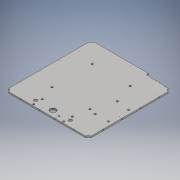
# Autodesk Inventor part: 001
Saved by Autodesk Inventor 2016 (Build 200138000, 138)
## iProperties
Created: 2015-10-17
Part Number: 001
Material: Generic
Document SubType Name: Modeling
Designer: iLyngklip
Density: 1 g/cm^3
Appearance: Default
Author: iLyngklip
Title: Mellemplade mk2
Autodesk Inventor part; units mm, degrees
ref_plane "YZ Plane" through (0, 0, 0) normal (1, 0, 0) x (0, 1, 0)
ref_plane "XZ Plane" through (0, 0, 0) normal (0, 1, 0) x (-1, 0, 0)
ref_plane "XY Plane" through (0, 0, 0) normal (0, 0, 1) x (1, 0, 0)
sketch "Sketch1" plane through (0, 0, 0) normal (0, 0, 1) x (1, 0, 0)
  line L0 (-154, 160) -> (154, 160)
  line L1 (154, 160) -> (154, -160)
  line L2 (154, -160) -> (-154, -160)
  line L3 (-154, -160) -> (-154, 160)
  point P0 (0, 0)
  dimension "d0" = 308
  dimension "d1" = 320
  dimension "d2" = 160
  dimension "d3" = 154
  constraints: 8 end point, 2 parallel, 1 horizontal, 1 perpendicular
  measures "d0" distance of L1.end L2.end
  measures "d1" distance of L0.end L1.end
  measures "d2" distance from line of L0 point (0, 0)
  measures "d3" distance from line of point (0, 0) L1
extrude "Tykkelse" add sketch "Sketch1" along normal blind 6
sketch "Sketch2" plane through (0, 0, 6) normal (0, 0, 1) x (1, 0, 0)
  circle A0 centre (65, -138) radius 6
  circle A1 centre (-65, -138) radius 6
  circle A2 centre (0, -138) radius 11
  line L0 (0, 0) -> (0, -168.7414) construction
  line L1 (-154, -160) -> (154, -160) projected
  line L2 (154, -160) -> (154, 160) projected
  dimension "d7" = 12
  dimension "d8" = 22
  dimension "d9" = 22
  dimension "d10" = 130
  dimension "d15" = 22
  dimension "d16" = 22
  dimension "d135" = 12
  dimension "d136" = 89
  constraints: 3 centre point, 2 end point, 1 point on line, 1 vertical
  measures "d7" diameter of A0
  measures "d8" diameter of A2
  measures "d9" distance from line of L1 A0.centre
  measures "d10" distance of A0.centre A1.centre
  measures "d15" distance from line of L1 A2.centre
  measures "d16" distance from line of L1 A1.centre
  measures "d135" diameter of A1
  measures "d136" distance from line of L2 A0.centre
extrude "Ø12 Glide hul" cut sketch "Sketch2" against normal blind 3 contours A0 | A1
extrude "Gevind hul" cut sketch "Sketch2" against normal blind 6 contours A2
sketch "Sketch3" plane through (0, 0, 6) normal (0, 0, 1) x (1, 0, 0)
  circle A0 centre (154, -160) radius 10
  line L0 (154, -160) -> (-154, -160) projected
  circle A1 centre (-154, -160) radius 10
  line L1 (154, 160) -> (-154, 160) projected
  circle A2 centre (154, 160) radius 11.5178
  circle A3 centre (-154, 160) radius 10
  point P0 (0, 0)
  dimension "d17" = 20
  dimension "d18" = 20
  dimension "d21" = 20
  dimension "d22" = 23.0357
  constraints: 4 centre point, 2 coincident
  measures "d17" diameter of A0
  measures "d18" diameter of A1
  measures "d21" diameter of A3
  measures "d22" diameter of A2
extrude "Ledningsrunding" cut sketch "Sketch3" against normal blind 10
sketch "Sketch4" plane through (0, 0, 0) normal (0, 0, -1) x (-1, 0, 0)
  circle A0 centre (56.15, -121.85) radius 1.5 projected
  circle A1 centre (56.15, -154.15) radius 1.5 projected
  circle A2 centre (-56.15, -154.15) radius 1.5 projected
  circle A3 centre (-56.15, -121.85) radius 1.5 projected
  point P0 (0, 0)
extrude "Step-spacer montering" cut sketch "Sketch4" against normal up to surface (6 mm away)
sketch "Sketch5" plane through (0, 0, 0) normal (0, 0, -1) x (-1, 0, 0)
  circle A0 centre (77, 85) radius 1.5
  circle A1 centre (77, -65) radius 1.5
  circle A2 centre (-65, -65) radius 1.5
  circle A3 centre (-65, 85) radius 1.5
  point P0 (0, 0)
  dimension "d119" = 3
  dimension "d120" = 150
  dimension "d121" = 142
  dimension "d122" = 85
  dimension "d123" = 65
  constraints: 4 centre point, 3 equal radius, 2 horizontal alignment, 2 vertical alignment
  measures "d119" diameter of A0
  measures "d120" distance of A1.centre A0.centre
  measures "d121" distance of A2.centre A1.centre
  measures "d122" vertical distance of point (0, 0) A0.centre
  measures "d123" horizontal distance of point (0, 0) A2.centre
extrude "PSU-Mount holes" cut sketch "Sketch5" against normal up to surface (6 mm away)
sketch "Sketch6" plane through (0, 0, 0) normal (0, 0, -1) x (-1, 0, 0)
  circle A0 centre (-90.74, -71.27) radius 1.5875 projected
  circle A1 centre (-139, -70) radius 1.5875 projected
  circle A2 centre (-139, 4.93) radius 1.5875 projected
  circle A3 centre (-90.74, 11.28) radius 1.5875 projected
  point P0 (0, 0)
extrude "Ramps Mount holes" cut sketch "Sketch6" against normal up to surface (6 mm away)
sketch "Sketch7" plane through (0, 0, 6) normal (0, 0, 1) x (1, 0, 0)
  line L0 (142.4822, 160) -> (-144, 160) projected
  line L1 (58.5, 160) -> (151.5, 160)
  line L2 (151.5, 160) -> (151.5, 152)
  line L3 (151.5, 152) -> (58.5, 152)
  line L4 (58.5, 152) -> (58.5, 160)
  line L5 (144.5, 166) -> (65.5, 166) projected
  line L6 (130.5, 152) -> (151.5, 152)
  line L7 (151.5, 152) -> (151.5, 148)
  line L8 (151.5, 148) -> (130.5, 148)
  line L9 (130.5, 148) -> (130.5, 152)
  line L10 (151.5, 148) -> (160.3981, 148)
  line L11 (160.3981, 148) -> (160.3981, 160)
  line L12 (160.3981, 160) -> (151.5, 160)
  line L13 (151.5, 160) -> (151.5, 148)
  point P0 (0, 0)
  dimension "d29" = 14
  dimension "d30" = 93
  dimension "d31" = 79
  dimension "d33" = 7
  dimension "d36" = 4
  dimension "d37" = 21
  constraints: 24 end point, 6 parallel, 3 horizontal, 3 perpendicular, 2 point on line
  measures "d29" distance between parallel lines of L3 L5
  measures "d30" distance of L2.end L3.end
  measures "d31" distance of L5.start L5.end
  measures "d33" horizontal distance of L5.end L3.end
  measures "d36" distance of L6.end L7.end
  measures "d37" distance of L7.end L8.end
extrude "Skærm-plads" cut sketch "Sketch7" against normal up to next
sketch "Sketch8" plane through (0, 0, 0) normal (0, 0, -1) x (-1, 0, 0)
  line L0 (-58.5, 160) -> (-58.5, 152) construction
  line L1 (-58.5, 152) -> (-130.5, 152) construction
  line L2 (-130.5, 152) -> (-130.5, 148) construction
  line L3 (-130.5, 148) -> (-154, 148) construction
  line L4 (-154, 148) -> (-154, -150) construction
  arc A0 (-144, -160) -> (-154, -150) centre (-154, -160) ccw construction
  line L5 (-144, -160) -> (144, -160) construction
  arc A1 (154, -150) -> (144, -160) centre (154, -160) ccw construction
  line L6 (154, -150) -> (154, 150) projected
  arc A2 (144, 160) -> (154, 150) centre (154, 160) ccw construction
  line L7 (144, 160) -> (-58.5, 160) projected
  circle A3 centre (0, -138) radius 11 construction
  circle A4 centre (56.15, -121.85) radius 1.5 construction
  circle A5 centre (56.15, -154.15) radius 1.5 construction
  circle A6 centre (-56.15, -121.85) radius 1.5 construction
  circle A7 centre (-56.15, -154.15) radius 1.5 construction
  circle A8 centre (-90.74, -71.27) radius 1.5875 construction
  circle A9 centre (-139, -70) radius 1.5875 construction
  circle A10 centre (-90.74, 11.28) radius 1.5875 construction
  circle A11 centre (-139, 4.93) radius 1.5875 construction
  line L8 (154, 103.5) -> (147.679, 103.5)
  line L9 (147.679, 103.5) -> (147.679, 103.5)
  line L10 (146.179, 102) -> (144.779, 102)
  line L11 (144.779, 108) -> (146.179, 108)
  line L12 (147.679, 106.5) -> (147.679, 106.5)
  line L13 (147.679, 106.5) -> (154, 106.5)
  arc A12 (146.179, 102) -> (147.679, 103.5) centre (146.179, 103.5) ccw
  arc A13 (147.679, 106.5) -> (146.179, 108) centre (146.179, 106.5) ccw
  arc A14 (143.279, 103.5) -> (144.779, 102) centre (144.779, 103.5) ccw
  arc A15 (143.279, 106.5) -> (143.279, 103.5) centre (143.279, 105) ccw
  arc A16 (143.279, 106.5) -> (142.4708, 103.7364) centre (143.279, 105) ccw
  arc A17 (144.779, 108) -> (143.279, 106.5) centre (144.779, 106.5) ccw
  line L14 (143.279, 105) -> (153.6341, 105) construction
  arc A18 (146.179, 32) -> (147.679, 33.5) centre (146.179, 33.5) ccw
  arc A19 (143.279, 33.5) -> (144.779, 32) centre (144.779, 33.5) ccw
  line L15 (146.179, 32) -> (144.779, 32)
  line L16 (154, 33.5) -> (147.679, 33.5)
  line L17 (147.679, 33.5) -> (147.679, 33.5)
  line L18 (147.679, 36.5) -> (154, 36.5)
  line L19 (147.679, 36.5) -> (147.679, 36.5)
  arc A20 (147.679, 36.5) -> (146.179, 38) centre (146.179, 36.5) ccw
  line L20 (143.279, 35) -> (153.6341, 35) construction
  line L21 (144.779, 38) -> (146.179, 38)
  arc A21 (143.279, 36.5) -> (143.279, 33.5) centre (143.279, 35) ccw
  arc A22 (143.279, 36.5) -> (142.4708, 33.7364) centre (143.279, 35) ccw
  arc A23 (144.779, 38) -> (143.279, 36.5) centre (144.779, 36.5) ccw
  arc A24 (146.179, -38) -> (147.679, -36.5) centre (146.179, -36.5) ccw
  arc A25 (143.279, -36.5) -> (144.779, -38) centre (144.779, -36.5) ccw
  line L22 (146.179, -38) -> (144.779, -38)
  line L23 (154, -36.5) -> (147.679, -36.5)
  line L24 (147.679, -36.5) -> (147.679, -36.5)
  line L25 (147.679, -33.5) -> (154, -33.5)
  line L26 (147.679, -33.5) -> (147.679, -33.5)
  arc A26 (147.679, -33.5) -> (146.179, -32) centre (146.179, -33.5) ccw
  line L27 (143.279, -35) -> (153.6341, -35) construction
  line L28 (144.779, -32) -> (146.179, -32)
  arc A27 (143.279, -33.5) -> (143.279, -36.5) centre (143.279, -35) ccw
  arc A28 (143.279, -33.5) -> (142.4708, -36.2636) centre (143.279, -35) ccw
  arc A29 (144.779, -32) -> (143.279, -33.5) centre (144.779, -33.5) ccw
  arc A30 (146.179, -108) -> (147.679, -106.5) centre (146.179, -106.5) ccw
  arc A31 (143.279, -106.5) -> (144.779, -108) centre (144.779, -106.5) ccw
  line L29 (146.179, -108) -> (144.779, -108)
  line L30 (154, -106.5) -> (147.679, -106.5)
  line L31 (147.679, -106.5) -> (147.679, -106.5)
  line L32 (147.679, -103.5) -> (154, -103.5)
  line L33 (147.679, -103.5) -> (147.679, -103.5)
  arc A32 (147.679, -103.5) -> (146.179, -102) centre (146.179, -103.5) ccw
  line L34 (143.279, -105) -> (153.6341, -105) construction
  line L35 (144.779, -102) -> (146.179, -102)
  arc A33 (143.279, -103.5) -> (143.279, -106.5) centre (143.279, -105) ccw
  arc A34 (143.279, -103.5) -> (142.4708, -106.2636) centre (143.279, -105) ccw
  arc A35 (144.779, -102) -> (143.279, -103.5) centre (144.779, -103.5) ccw
  line L36 (144, -160) -> (-144, -160) projected
  line L37 (100.5, -160) -> (100.5, -153.679)
  line L38 (97.5, -160) -> (97.5, -153.679)
  arc A36 (100.5, -149.279) -> (97.5, -149.279) centre (99, -149.279) ccw
  arc A37 (96, -152.179) -> (97.5, -153.679) centre (97.5, -152.179) ccw
  line L39 (96, -152.179) -> (96, -150.779)
  arc A38 (97.5, -149.279) -> (96, -150.779) centre (97.5, -150.779) ccw
  arc A39 (100.5, -153.679) -> (102, -152.179) centre (100.5, -152.179) ccw
  line L40 (102, -152.179) -> (102, -150.779)
  arc A40 (102, -150.779) -> (100.5, -149.279) centre (100.5, -150.779) ccw
  line L41 (26, -152.179) -> (26, -150.779)
  arc A41 (27.5, -149.279) -> (26, -150.779) centre (27.5, -150.779) ccw
  arc A42 (26, -152.179) -> (27.5, -153.679) centre (27.5, -152.179) ccw
  arc A43 (30.5, -149.279) -> (27.5, -149.279) centre (29, -149.279) ccw
  line L42 (27.5, -160) -> (27.5, -153.679)
  arc A44 (32, -150.779) -> (30.5, -149.279) centre (30.5, -150.779) ccw
  line L43 (32, -152.179) -> (32, -150.779)
  arc A45 (30.5, -153.679) -> (32, -152.179) centre (30.5, -152.179) ccw
  line L44 (30.5, -160) -> (30.5, -153.679)
  line L45 (99, -149.279) -> (99, -156.2509) construction
  line L46 (-67.1744, 0) -> (89.9011, 0) construction
  line L47 (0, -73.7565) -> (0, 76.0519) construction
  line L48 (100.5, 160) -> (100.5, 153.679)
  line L49 (97.5, 160) -> (97.5, 153.679)
  arc A46 (97.5, 149.279) -> (100.5, 149.279) centre (99, 149.279) ccw
  arc A47 (97.5, 153.679) -> (96, 152.179) centre (97.5, 152.179) ccw
  line L50 (96, 152.179) -> (96, 150.779)
  arc A48 (96, 150.779) -> (97.5, 149.279) centre (97.5, 150.779) ccw
  arc A49 (102, 152.179) -> (100.5, 153.679) centre (100.5, 152.179) ccw
  line L51 (102, 152.179) -> (102, 150.779)
  arc A50 (100.5, 149.279) -> (102, 150.779) centre (100.5, 150.779) ccw
  line L52 (99, 149.279) -> (99, 156.2509) construction
  arc A51 (-1.5, 149.279) -> (1.5, 149.279) centre (0, 149.279) ccw
  arc A52 (-3, 150.779) -> (-1.5, 149.279) centre (-1.5, 150.779) ccw
  arc A53 (1.5, 149.279) -> (3, 150.779) centre (1.5, 150.779) ccw
  line L53 (-3, 152.179) -> (-3, 150.779)
  line L54 (3, 152.179) -> (3, 150.779)
  arc A54 (-1.5, 153.679) -> (-3, 152.179) centre (-1.5, 152.179) ccw
  arc A55 (3, 152.179) -> (1.5, 153.679) centre (1.5, 152.179) ccw
  line L55 (0, 149.279) -> (0, 156.2509) construction
  line L56 (-1.5, 160) -> (-1.5, 153.679)
  line L57 (1.5, 160) -> (1.5, 153.679)
  arc A56 (-147.679, 33.5) -> (-146.179, 32) centre (-146.179, 33.5) ccw
  arc A57 (-144.779, 32) -> (-143.279, 33.5) centre (-144.779, 33.5) ccw
  line L58 (-146.179, 32) -> (-144.779, 32)
  line L59 (-154, 33.5) -> (-147.679, 33.5)
  line L60 (-147.679, 33.5) -> (-147.679, 33.5)
  line L61 (-147.679, 36.5) -> (-154, 36.5)
  line L62 (-147.679, 36.5) -> (-147.679, 36.5)
  arc A58 (-146.179, 38) -> (-147.679, 36.5) centre (-146.179, 36.5) ccw
  line L63 (-143.279, 35) -> (-153.6341, 35) construction
  line L64 (-144.779, 38) -> (-146.179, 38)
  arc A59 (-143.279, 33.5) -> (-143.279, 36.5) centre (-143.279, 35) ccw
  arc A60 (-142.4708, 33.7364) -> (-143.279, 36.5) centre (-143.279, 35) ccw
  arc A61 (-143.279, 36.5) -> (-144.779, 38) centre (-144.779, 36.5) ccw
  arc A62 (-143.279, -36.5) -> (-143.279, -33.5) centre (-143.279, -35) ccw
  arc A63 (-142.4708, -36.2636) -> (-143.279, -33.5) centre (-143.279, -35) ccw
  arc A64 (-144.779, -38) -> (-143.279, -36.5) centre (-144.779, -36.5) ccw
  line L65 (-144.779, -32) -> (-146.179, -32)
  arc A65 (-143.279, -33.5) -> (-144.779, -32) centre (-144.779, -33.5) ccw
  line L66 (-146.179, -38) -> (-144.779, -38)
  arc A66 (-147.679, -36.5) -> (-146.179, -38) centre (-146.179, -36.5) ccw
  line L67 (-147.679, -36.5) -> (-147.679, -36.5)
  line L68 (-147.679, -33.5) -> (-147.679, -33.5)
  arc A67 (-146.179, -32) -> (-147.679, -33.5) centre (-146.179, -33.5) ccw
  line L69 (-143.279, -35) -> (-153.6341, -35) construction
  line L70 (-154, -36.5) -> (-147.679, -36.5)
  line L71 (-147.679, -33.5) -> (-154, -33.5)
  arc A68 (-143.279, -106.5) -> (-143.279, -103.5) centre (-143.279, -105) ccw
  arc A69 (-142.4708, -106.2636) -> (-143.279, -103.5) centre (-143.279, -105) ccw
  arc A70 (-144.779, -108) -> (-143.279, -106.5) centre (-144.779, -106.5) ccw
  line L72 (-144.779, -102) -> (-146.179, -102)
  arc A71 (-143.279, -103.5) -> (-144.779, -102) centre (-144.779, -103.5) ccw
  line L73 (-146.179, -108) -> (-144.779, -108)
  arc A72 (-147.679, -106.5) -> (-146.179, -108) centre (-146.179, -106.5) ccw
  line L74 (-147.679, -106.5) -> (-147.679, -106.5)
  line L75 (-147.679, -103.5) -> (-147.679, -103.5)
  arc A73 (-146.179, -102) -> (-147.679, -103.5) centre (-146.179, -103.5) ccw
  line L76 (-143.279, -105) -> (-153.6341, -105) construction
  line L77 (-154, -106.5) -> (-147.679, -106.5)
  line L78 (-147.679, -103.5) -> (-154, -103.5)
  line L79 (-100.5, -160) -> (-100.5, -153.679)
  line L80 (-97.5, -160) -> (-97.5, -153.679)
  arc A74 (-97.5, -149.279) -> (-100.5, -149.279) centre (-99, -149.279) ccw
  arc A75 (-97.5, -153.679) -> (-96, -152.179) centre (-97.5, -152.179) ccw
  line L81 (-96, -152.179) -> (-96, -150.779)
  arc A76 (-96, -150.779) -> (-97.5, -149.279) centre (-97.5, -150.779) ccw
  arc A77 (-102, -152.179) -> (-100.5, -153.679) centre (-100.5, -152.179) ccw
  line L82 (-102, -152.179) -> (-102, -150.779)
  arc A78 (-100.5, -149.279) -> (-102, -150.779) centre (-100.5, -150.779) ccw
  line L83 (-26, -152.179) -> (-26, -150.779)
  arc A79 (-26, -150.779) -> (-27.5, -149.279) centre (-27.5, -150.779) ccw
  arc A80 (-27.5, -153.679) -> (-26, -152.179) centre (-27.5, -152.179) ccw
  arc A81 (-27.5, -149.279) -> (-30.5, -149.279) centre (-29, -149.279) ccw
  line L84 (-27.5, -160) -> (-27.5, -153.679)
  arc A82 (-30.5, -149.279) -> (-32, -150.779) centre (-30.5, -150.779) ccw
  line L85 (-32, -152.179) -> (-32, -150.779)
  arc A83 (-32, -152.179) -> (-30.5, -153.679) centre (-30.5, -152.179) ccw
  line L86 (-30.5, -160) -> (-30.5, -153.679)
  line L87 (-99, -149.279) -> (-99, -156.2509) construction
  line L88 (-154, -150) -> (-154, 148.4822) projected
  line L89 (-154, 103.5) -> (-147.679, 103.5)
  line L90 (-154, 106.4661) -> (-147.679, 106.4661)
  arc A84 (-147.679, 103.5) -> (-146.1791, 102) centre (-146.179, 103.5) ccw
  line L91 (-146.1791, 102) -> (-144.7791, 102)
  arc A85 (-144.7791, 102) -> (-143.2791, 103.5) centre (-144.7791, 103.5) ccw
  arc A86 (-143.2791, 103.5) -> (-143.2791, 106.5) centre (-143.2791, 105) ccw
  arc A87 (-143.2791, 106.5) -> (-144.7787, 107.9661) centre (-144.7787, 106.4661) ccw
  arc A88 (-146.1787, 107.9661) -> (-147.679, 106.4661) centre (-146.179, 106.4661) ccw
  line L92 (-146.1787, 107.9661) -> (-144.7787, 107.9661)
  line L93 (-143.2791, 105) -> (-148.8776, 105) construction
  line L94 (154, 106.5) -> (154, 103.5)
  line L95 (154, 36.5) -> (154, 33.5)
  line L96 (154, 150) -> (154, -150) projected
  line L97 (154, -33.5) -> (154, -36.5)
  line L98 (154, -103.5) -> (154, -106.5)
  line L99 (100.5, -160) -> (97.5, -160)
  line L100 (30.5, -160) -> (27.5, -160)
  line L101 (-27.5, -160) -> (-30.5, -160)
  line L102 (-97.5, -160) -> (-100.5, -160)
  line L103 (-154, -106.5) -> (-154, -103.5)
  line L104 (-154, -36.5) -> (-154, -33.5)
  line L105 (-154, 33.5) -> (-154, 36.5)
  line L106 (-154, 103.5) -> (-154, 106.4661)
  line L107 (100.5, 160) -> (97.5, 160)
  line L108 (144, 160) -> (-58.5, 160) projected
  line L109 (1.5, 160) -> (-1.5, 160)
  point P0 (0, 0)
  point P1 (147.679, 106.5)
  point P2 (143.279, 33.5)
  point P3 (147.679, 36.5)
  point P4 (147.679, -33.5)
  point P5 (147.679, -103.5)
  point P6 (-143.279, 33.5)
  point P7 (-147.679, 36.5)
  point P8 (-143.279, -36.5)
  point P9 (-147.679, -33.5)
  point P10 (-147.679, -103.5)
  dimension "d38" = 6.321
  dimension "d40" = 1.5
  dimension "d41" = 1.4
  dimension "d42" = 1.5
  dimension "d43" = 1.5
  dimension "d44" = 1.4
  dimension "d45" = 55
  dimension "d48" = 70
  dimension "d56" = 1.5
  dimension "d57" = 1.4
  dimension "d58" = 1.5
  dimension "d59" = 6.321
  dimension "d60" = 1.5
  dimension "d61" = 1.4
  dimension "d62" = 1.5
  dimension "d63" = 1.5
  dimension "d66" = 70
  dimension "d71" = 55
  dimension "d74" = 99
  dimension "d81" = 70
  dimension "d86" = 1.5
  dimension "d87" = 1.4
  dimension "d88" = 6.321
  dimension "d91" = 55
  constraints: 203 end point, 160 point on circle, 77 centre point, 70 symmetric about line, 27 point on line, 21 coincident, 16 vertical, 12 collinear, 12 horizontal alignment, 11 tangent, 10 perpendicular, 9 horizontal, 7 equal radius, 7 vertical alignment, 4 parallel, 1 midpoint, 281 other
  measures "d38" distance of L8.start L8.end
  measures "d40" radius of A12
  measures "d41" distance of L11.start L11.end
  measures "d42" radius of A15
  measures "d43" radius of A17
  measures "d44" distance of A17.centre A13.centre
  measures "d45" distance between parallel lines of L7 L14
  measures "d48" distance of A12.centre A18.centre
  measures "d56" radius of A37
  measures "d57" distance of L39.start L39.end
  measures "d58" radius of A38
  measures "d59" distance of L38.start L38.end
  measures "d60" radius of A39
  measures "d61" distance of L40.start L40.end
  measures "d62" radius of A40
  measures "d63" radius of A36
  measures "d66" distance of L39.start L41.start
  measures "d71" distance between parallel lines of L6 L45
  measures "d74" distance of L52.start L55.start
  measures "d81" distance of A60.start A63.start
  measures "d86" radius of A88
  measures "d87" distance of L91.start L91.end
  measures "d88" distance of L89.start L89.end
  measures "d91" distance between parallel lines of L7 L93
extrude "Monteringshuller" cut sketch "Sketch8" against normal blind 5
sketch "Sketch10" plane through (0, 0, 6) normal (0, 0, 1) x (1, 0, 0)
  line L0 (58.5, 152) -> (58.5, 160) projected
  line L1 (58.5, 160) -> (-144, 160) projected
  arc A0 (-154, 150) -> (-144, 160) centre (-154, 160) ccw projected
  line L2 (-154, 150) -> (-154, -150) projected
  arc A1 (-144, -160) -> (-154, -150) centre (-154, -160) ccw projected
  line L3 (-144, -160) -> (144, -160) projected
  arc A2 (154, -150) -> (144, -160) centre (154, -160) ccw projected
  line L4 (154, -150) -> (154, 148) projected
  line L5 (154, 148) -> (130.5, 148) projected
  line L6 (130.5, 148) -> (130.5, 152) projected
  line L7 (130.5, 152) -> (58.5, 152) projected
  circle A3 centre (139, 4.93) radius 1.5875 projected
  circle A4 centre (90.74, 11.28) radius 1.5875 projected
  circle A5 centre (139, -70) radius 1.5875 projected
  circle A6 centre (90.74, -71.27) radius 1.5875 projected
  circle A7 centre (56.15, -154.15) radius 1.5 projected
  circle A8 centre (56.15, -121.85) radius 1.5 projected
  circle A9 centre (-56.15, -154.15) radius 1.5 projected
  circle A10 centre (-56.15, -121.85) radius 1.5 projected
  circle A11 centre (0, -138) radius 11 projected
  circle A12 centre (65, -138) radius 6 projected
  circle A13 centre (-65, -138) radius 6 projected
  circle A14 centre (139, -70) radius 3.5
  circle A15 centre (90.74, -71.27) radius 3.5
  circle A16 centre (90.74, 11.28) radius 3.5
  circle A17 centre (139, 4.93) radius 3.5
  circle A18 centre (-56.15, -121.85) radius 3.5
  circle A19 centre (-56.15, -154.15) radius 3.5
  circle A20 centre (56.15, -154.15) radius 3.5
  circle A21 centre (56.15, -121.85) radius 3.5
  circle A22 centre (-77, 85) radius 1.5 projected
  circle A23 centre (-77, 85) radius 1.5 projected
  circle A24 centre (65, 85) radius 1.5 projected
  circle A25 centre (65, 85) radius 1.5 projected
  circle A26 centre (65, -65) radius 1.5 projected
  circle A27 centre (65, -65) radius 1.5 projected
  circle A28 centre (-77, -65) radius 1.5 projected
  circle A29 centre (-77, -65) radius 1.5 projected
  circle A30 centre (-77, 85) radius 3.5
  circle A31 centre (65, 85) radius 3.5
  circle A32 centre (65, -65) radius 3.5
  circle A33 centre (-77, -65) radius 3.5
  point P0 (0, 0)
  dimension "d137" = 7
  dimension "d138" = 7
  dimension "d139" = 7
  constraints: 12 centre point, 9 equal radius
  measures "d137" diameter of A14
  measures "d138" diameter of A18
  measures "d139" diameter of A33
extrude "Undersænkning af skruehoveder" cut sketch "Sketch10" against normal blind 3 contours A14 | A15 | A16 | A17 | A18 | A19 | A20 | A21 | A22 | A24 | A30 | A31 | A32 | A33
sketch "Sketch11" plane through (0, 0, 6) normal (0, 0, 1) x (1, 0, 0)
  arc A0 (109.0858, 152) -> (110.5, 150) centre (110.5, 151.5) ccw
  line L0 (110.5, 150) -> (130.5, 150)
  line L1 (130.5, 152) -> (58.5, 152) projected
  line L2 (130.5, 148) -> (130.5, 152) projected
  arc A1 (79.0858, 152) -> (80.5, 150) centre (80.5, 151.5) ccw
  arc A2 (97.5, 150) -> (98.9142, 152) centre (97.5, 151.5) ccw
  line L3 (97.5, 150) -> (80.5, 150)
  circle A3 centre (154, 148) radius 10
  arc A4 (154, -150) -> (144, -160) centre (154, -160) ccw projected
  point P0 (0, 0)
  dimension "d108" = 3
  dimension "d109" = 2
  dimension "d110" = 20
  dimension "d111" = 3
  dimension "d112" = 17
  dimension "d113" = 2
  dimension "d114" = 13
  dimension "d117" = 10
  dimension "d118" = 20
  constraints: 6 point on circle, 4 centre point, 4 end point, 3 point on line, 3 tangent, 2 parallel, 1 equal radius, 1 midpoint
  measures "d108" diameter of A0
  measures "d109" distance between parallel lines of L1 L0
  measures "d110" horizontal distance of L0.end A0.centre
  measures "d111" diameter of A1
  measures "d112" distance of A1.centre A2.centre
  measures "d113" distance between parallel lines of L1 L3
  measures "d114" distance of A0.centre A2.centre
  measures "d117" radius of A4
  measures "d118" diameter of A3
extrude "Ledningshul v. skærm" cut sketch "Sketch11" against normal up to surface (6 mm away)
sketch "Sketch12" plane through (0, 0, 6) normal (0, 0, 1) x (1, 0, 0)
  arc A0 (32, -146.5) -> (32, -143.5) centre (32, -145) ccw
  arc A1 (27, -143.5) -> (27, -146.5) centre (27, -145) ccw
  line L0 (27, -146.5) -> (32, -146.5)
  line L1 (27, -143.5) -> (32, -143.5)
  line L2 (-144, -160) -> (144, -160) projected
  line L3 (154, -150) -> (154, 138) projected
  point P0 (0, 0)
  dimension "d128" = 3
  dimension "d130" = 5
  dimension "d131" = 15
  dimension "d132" = 122
  constraints: 4 end point, 4 point on circle, 4 tangent, 2 centre point, 1 equal radius, 1 horizontal alignment
  measures "d128" diameter of A0
  measures "d130" distance of A0.centre A1.centre
  measures "d131" distance from line of L2 A0.centre
  measures "d132" distance from line of L3 A0.centre
extrude "Ledningshul v. Z-stop" cut sketch "Sketch12" against normal up to surface (6 mm away)
fillet "Fillet1" radius 1.5 1 edges at (58.5, 152, 3)
equation "\"d2\" = 0.5 * d1"
equation "\"d3\" = 0.5 * d0"
equation "\"d15\" = d9"
equation "\"d16\" = d9"
equation "\"d18\" = d17"
equation "\"d21\" = d17"
equation "\"d33\" = -0.5 * d31 + 0.5 * d30"
equation "\"d81\" = d48"
equation "\"d91\" = d45"
body "Solid1"
